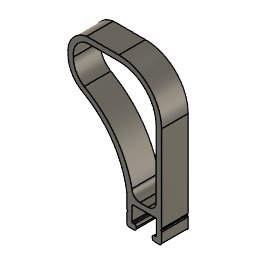
Refuerzo (Autodesk Fusion 360 design; units mm, degrees)
part number: 2025-12-28-18-20-55-018
Autodesk Fusion 360 part; units mm, degrees
sketch "Boceto1" plane through (0, 0, 0) normal (0, 1, 0) x (1, 0, 0)
  line L0 (0, 0) -> (22.1, 0) construction
  line L1 (22.8, 0) -> (24.95, 0)
  line L2 (25.65, -0.7) -> (25.65, -1.3)
  line L3 (24.95, -2) -> (24.3025, -2)
  line L4 (24.0025, -2.3025) -> (24.0475, -7.6525)
  line L5 (24.3475, -7.95) -> (32.85, -7.95)
  line L6 (33.15, -7.65) -> (33.15, -2.3)
  line L7 (32.85, -2) -> (32.25, -2)
  line L8 (31.55, -1.3) -> (31.55, -0.7)
  line L9 (32.25, 0) -> (34.4, 0)
  line L10 (35.1, -0.7) -> (35.1, -4.4424)
  line L11 (34.9021, -4.8649) -> (34.8, -4.95)
  line L12 (34.8, -4.95) -> (34.9725, -5.157)
  line L13 (35.1, -5.5091) -> (35.1, -38)
  line L14 (19.1, -54) -> (7, -54)
  line L15 (22.1, -0.7) -> (22.1, -4.4548)
  line L16 (22.2823, -4.8639) -> (22.4059, -4.975)
  line L17 (22.4059, -4.975) -> (22.241, -5.1585)
  line L18 (22.1, -5.5262) -> (22.1, -10.4)
  arc A0 (22.1, -4.4548) -> (22.2823, -4.8639) centre (22.65, -4.4548) ccw
  arc A1 (22.241, -5.1585) -> (22.1, -5.5262) centre (22.65, -5.5262) ccw
  arc A2 (35.1, -5.5091) -> (34.9725, -5.157) centre (34.55, -5.5091) ccw
  arc A3 (34.9021, -4.8649) -> (35.1, -4.4424) centre (34.55, -4.4424) ccw
  arc A4 (24.95, -2) -> (25.65, -1.3) centre (24.95, -1.3) ccw
  arc A5 (25.65, -0.7) -> (24.95, 0) centre (24.95, -0.7) ccw
  arc A6 (22.8, 0) -> (22.1, -0.7) centre (22.8, -0.7) ccw
  arc A7 (31.55, -1.3) -> (32.25, -2) centre (32.25, -1.3) ccw
  arc A8 (32.25, 0) -> (31.55, -0.7) centre (32.25, -0.7) ccw
  arc A9 (35.1, -0.7) -> (34.4, 0) centre (34.4, -0.7) ccw
  arc A10 (24.3025, -2) -> (24.0025, -2.3025) centre (24.3025, -2.3) ccw
  arc A11 (33.15, -2.3) -> (32.85, -2) centre (32.85, -2.3) ccw
  arc A12 (24.0475, -7.6525) -> (24.3475, -7.95) centre (24.3475, -7.65) ccw
  arc A13 (32.85, -7.95) -> (33.15, -7.65) centre (32.85, -7.65) ccw
  arc A14 (19.1, -54) -> (35.1, -38) centre (19.1, -38) ccw
  arc A15 (5, -35.5) -> (22.1, -10.4) centre (-10.943, -6.2635) ccw
  arc A16 (5, -35.5) -> (0, -44.75) centre (10.5938, -44.5) ccw
  arc A17 (0, -44.75) -> (7, -54) centre (8.3384, -45.7135) ccw
  line L19 (19.1, -51.9418) -> (7.1768, -51.9418)
  arc A18 (2.0623, -44.8467) -> (7.1768, -51.9418) centre (8.3384, -45.7135) ccw
  arc A19 (6.0739, -37.2559) -> (2.0623, -44.8467) centre (10.5938, -44.5) ccw
  line L20 (33.0418, -13.1919) -> (33.0418, -38)
  arc A20 (19.1, -51.9418) -> (33.0418, -38) centre (19.1, -38) ccw
  line L21 (33.0418, -13.1919) -> (33.0418, -13)
  line L22 (30.0418, -10) -> (27, -10)
  arc A21 (27, -10) -> (24, -13) centre (27, -13) ccw
  arc A22 (33.0418, -13) -> (30.0418, -10) centre (30.0418, -13) ccw
  arc A23 (6.0739, -37.2559) -> (24, -13) centre (-11.3447, -5.6309) ccw
  dimension "d1" = 0.55
  dimension "d2" = 0.7
  dimension "d3" = 0.3
  dimension "d4" = 0.3
  dimension "d5" = 16
  dimension "d9" = 3
  constraint coincident L0.start origin
  constraint horizontal L0
  constraint parallel L0 L1
  constraint perpendicular L1 L2
  constraint perpendicular L2 L3
  constraint perpendicular L2 L5
  constraint perpendicular L5 L6
  constraint perpendicular L6 L7
  constraint perpendicular L7 L8
  constraint perpendicular L8 L9
  constraint perpendicular L9 L10
  constraint perpendicular L11 L12
  constraint perpendicular L5 L13
  constraint perpendicular L13 L14
  constraint perpendicular L0 L15
  constraint perpendicular L16 L17
  constraint parallel L15 L18
  constraint tangent L15 A0
  constraint tangent L16 A0
  constraint tangent L17 A1
  constraint tangent L18 A1
  constraint equal A0 A1
  constraint tangent L12 A2
  constraint tangent L13 A2
  constraint equal A0 A2
  constraint tangent L10 A3
  constraint tangent L11 A3
  constraint equal A0 A3
  constraint tangent L2 A4
  constraint tangent L3 A4
  constraint tangent L1 A5
  constraint tangent L2 A5
  constraint equal A4 A5
  constraint coincident L0.end L15
  constraint coincident L0.end L1
  constraint tangent L15 A6
  constraint tangent L1 A6
  constraint equal A4 A6
  constraint tangent L7 A7
  constraint tangent L8 A7
  constraint equal A4 A7
  constraint tangent L8 A8
  constraint tangent L9 A8
  constraint equal A4 A8
  constraint tangent L9 A9
  constraint tangent L10 A9
  constraint equal A4 A9
  constraint tangent L3 A10
  constraint tangent L4 A10
  constraint tangent L6 A11
  constraint tangent L7 A11
  constraint equal A10 A11
  constraint tangent L4 A12
  constraint tangent L5 A12
  constraint tangent L5 A13
  constraint tangent L6 A13
  constraint equal A12 A13
  constraint tangent L13 A14
  constraint tangent L14 A14
  constraint concentric A17 A18
  constraint concentric A16 A19
  constraint concentric A14 A20
  constraint tangent L19 A20
  constraint tangent L20 A20
  constraint parallel L20 L21
  constraint perpendicular L21 L22
  constraint tangent L22 A21
  constraint tangent L21 A22
  constraint tangent L22 A22
  constraint equal A21 A22
  measures "d1" radius of A0
  measures "d2" radius of A4
  measures "d3" radius of A10
  measures "d4" radius of A12
  measures "d5" radius of A14
  measures "d9" radius of A21
extrude "Extruir1" add sketch "Boceto1" along normal blind 10
equation "L = 10 mm"
equation "d11 = L"
